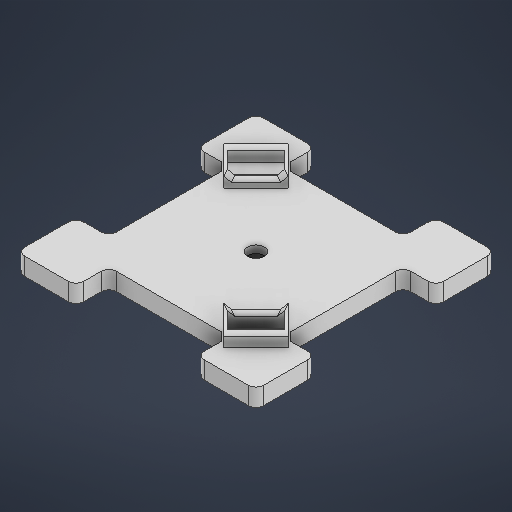
# Autodesk Inventor part: SistemaDeDesacople
Saved by Autodesk Inventor 2026.1 (Build 301233000, 233)
## iProperties
Created: 2026-01-17
Part Number: SistemaDeDesacople
Material: Genérico
Document SubType Name: Modeling
Designer: vickh
Density: 1 g/cm^3
Appearance: Valor por defecto
Author: vickh
Autodesk Inventor part; units mm, degrees
ref_plane "YZ Plane" through (0, 0, 0) normal (1, 0, 0) x (0, 1, 0)
ref_plane "XZ Plane" through (0, 0, 0) normal (0, 1, 0) x (-1, 0, 0)
ref_plane "XY Plane" through (0, 0, 0) normal (0, 0, 1) x (1, 0, 0)
sketch "Boceto1" plane through (0, 0, 0) normal (0, 1, 0) x (-1, 0, 0)
  line L0 (34.5, 0) -> (34.5, 24)
  line L1 (34.5, 24) -> (47.5, 24)
  line L2 (24, 47.5) -> (24, 34.5)
  line L3 (24, 34.5) -> (-24, 34.5)
  line L4 (-24, 34.5) -> (-24, 47.5)
  line L5 (-34.5, 24) -> (-47.5, 24)
  line L6 (47.5, 0) -> (-47.5, 0) construction
  line L7 (-47.5, 47.5) -> (-24, 47.5)
  line L8 (24, 47.5) -> (47.5, 47.5)
  line L9 (-47.5, 24) -> (-47.5, 47.5)
  line L10 (47.5, 47.5) -> (47.5, 24)
  line L11 (-34.5, 24) -> (-34.5, 0)
  line L12 (34.5, 0) -> (34.5, -24)
  line L13 (34.5, -24) -> (47.5, -24)
  line L14 (24, -47.5) -> (24, -34.5)
  line L15 (24, -34.5) -> (-24, -34.5)
  line L16 (-24, -34.5) -> (-24, -47.5)
  line L17 (-34.5, -24) -> (-47.5, -24)
  line L18 (-47.5, -47.5) -> (-24, -47.5)
  line L19 (24, -47.5) -> (47.5, -47.5)
  line L20 (-47.5, -24) -> (-47.5, -47.5)
  line L21 (47.5, -47.5) -> (47.5, -24)
  line L22 (-34.5, -24) -> (-34.5, 0)
  line L23 (-47.5, -47.5) -> (47.5, 47.5) construction
  line L24 (-47.5, 47.5) -> (47.5, -47.5) construction
  point P0 (0, 0)
  point P1 (0, -34.5)
  point P2 (24, 41)
  point P3 (0, 0)
  point P4 (35.75, 47.5)
  dimension "d0" = 95
  dimension "d9" = 13
  dimension "d10" = 23.5
  dimension "d15" = 23.5
  dimension "d71" = 95
  constraints: 50 end point, 10 symmetric about line, 6 perpendicular, 5 midpoint, 4 equal length, 3 vertical, 2 point on line, 1 coincident, 1 horizontal, 1 parallel
  measures "d0" distance of L7.start L8.end
  measures "d9" distance from line of L2.start L3
  measures "d10" distance between parallel lines of L9 L4
  measures "d15" distance of L5.end L7.start
  measures "d71" distance from line of point (35.75, 47.5) L19
extrude "Extrusión1" add sketch "Boceto1" along normal blind 7
chamfer "Chaflán4" distance 3.2 angle 45 4 edges at (24, 3.5, 34.5) (34.5, 3.5, 24) (-24, 3.5, -34.5) (-34.5, 3.5, -24)
sketch "Boceto2" plane through (0, 7, 0) normal (0, 1, 0) x (1, 0, 0)
  line L0 (-27.5, -27.5) -> (27.5, -27.5)
  line L1 (27.5, -27.5) -> (27.5, 27.5)
  line L2 (27.5, 27.5) -> (-27.5, 27.5)
  line L3 (-27.5, 27.5) -> (-27.5, -27.5)
  line L4 (-27.5, -27.5) -> (27.5, 27.5) construction
  line L5 (27.5, -27.5) -> (-27.5, 27.5) construction
  line L6 (-29.9749, 18.6612) -> (-18.6612, 29.9749)
  line L7 (-18.6612, 29.9749) -> (-25.0251, 36.3388)
  line L8 (-25.0251, 36.3388) -> (-36.3388, 25.0251)
  line L9 (-36.3388, 25.0251) -> (-29.9749, 18.6612)
  line L10 (-29.9749, 18.6612) -> (-25.0251, 36.3388) construction
  line L11 (-18.6612, 29.9749) -> (-36.3388, 25.0251) construction
  line L12 (-15.4792, 28.2071) -> (-26.7929, 39.5208)
  line L13 (-26.7929, 39.5208) -> (-39.5208, 26.7929)
  line L14 (-39.5208, 26.7929) -> (-28.2071, 15.4792)
  line L15 (-28.2071, 15.4792) -> (-15.4792, 28.2071)
  line L16 (-15.4792, 28.2071) -> (-39.5208, 26.7929) construction
  line L17 (-26.7929, 39.5208) -> (-28.2071, 15.4792) construction
  line L18 (-34.5, 24) -> (-34.5, -24) projected
  line L19 (-34.5, 0) -> (34.5, 0) construction
  line L20 (34.5, -24) -> (34.5, 24) projected
  line L21 (-18.6612, 29.9749) -> (-15.4792, 28.2071)
  line L22 (-29.9749, 18.6612) -> (-28.2071, 15.4792)
  line L23 (29.9749, -18.6612) -> (18.6612, -29.9749)
  line L24 (18.6612, -29.9749) -> (36.3388, -25.0251) construction
  line L25 (18.6612, -29.9749) -> (15.4792, -28.2071)
  line L26 (15.4792, -28.2071) -> (39.5208, -26.7929) construction
  line L27 (25.0251, -36.3388) -> (36.3388, -25.0251)
  line L28 (29.9749, -18.6612) -> (25.0251, -36.3388) construction
  line L29 (18.6612, -29.9749) -> (25.0251, -36.3388)
  line L30 (26.7929, -39.5208) -> (28.2071, -15.4792) construction
  line L31 (15.4792, -28.2071) -> (26.7929, -39.5208)
  line L32 (26.7929, -39.5208) -> (39.5208, -26.7929)
  line L33 (28.2071, -15.4792) -> (15.4792, -28.2071)
  line L34 (36.3388, -25.0251) -> (29.9749, -18.6612)
  line L35 (29.9749, -18.6612) -> (28.2071, -15.4792)
  line L36 (39.5208, -26.7929) -> (28.2071, -15.4792)
  point P0 (0, 0)
  point P1 (-27.5, 27.5)
  point P2 (27.5, -27.5)
  point P3 (27.5, -27.5)
  point P4 (34.5, -24)
  dimension "d21" = 55
  dimension "d22" = 55
  dimension "d23" = 16
  dimension "d24" = 9
  dimension "d25" = 18
  dimension "d26" = 16
  dimension "d51" = 135
  dimension "d52" = 135
  dimension "d55" = 360
  constraints: 70 end point, 11 midpoint, 6 parallel, 3 perpendicular, 2 horizontal, 51 other
  measures "d21" distance of L2.end L1.end
  measures "d22" distance of L1.end L0.end
  measures "d23" distance of L8.end L7.end
  measures "d24" distance of L7.end L6.end
  measures "d25" distance of L12.end L13.end
  measures "d26" distance of L13.end L14.end
  measures "d51" angle of L12 L2
  measures "d52" angle of L7 L2
sketch "Boceto3" plane through (0, 0, 0) normal (0, -1, 0) x (1, 0, 0)
  line L0 (47.5, 47.5) -> (47.5, 24) projected
  line L1 (47.5, 47.5) -> (24, 47.5)
  line L2 (24, 47.5) -> (24, 24)
  line L3 (24, 24) -> (47.5, 24)
  line L4 (47.5, 24) -> (47.5, 47.5)
  line L5 (24, 34.5) -> (24, 47.5) projected
  line L6 (47.5, 24) -> (34.5, 24) projected
  circle A0 centre (40.75, 40.75) radius 2.5
  line L7 (0, 48.9307) -> (0, -48.9307) construction
  line L8 (51.06, 0) -> (-51.06, 0) construction
  circle A1 centre (-40.75, 40.75) radius 2.5
  circle A2 centre (-40.75, -40.75) radius 2.5
  circle A3 centre (40.75, -40.75) radius 2.5
  line L9 (47.5, 47.5) -> (24, 24) construction
  line L10 (24, 47.5) -> (47.5, 24) construction
  point P0 (0, 0)
  point P1 (0, 0)
  point P2 (35.75, 35.75)
  dimension "d41" = 5
  dimension "d77" = 360
  dimension "d80" = 5
  constraints: 16 end point, 4 centre point, 3 midpoint, 2 collinear, 2 horizontal, 2 parallel, 1 coincident, 1 perpendicular, 1 point on line, 1 vertical, 9 other
  measures "d41" diameter of A0
  measures "d80" horizontal distance of A0.centre point (35.75, 35.75)
extrude "Extrusión6" cut sketch "Boceto3" against normal blind 4 contours A0 | A1 | A2 | A3
sketch "Boceto4" plane through (0, 7, 0) normal (0, 1, 0) x (1, 0, 0)
  circle A0 centre (0, 0) radius 3.3
  dimension "d44" = 6.6
  constraints: 1 centre point, 1 coincident
  measures "d44" diameter of A0
extrude "Extrusión7" cut sketch "Boceto4" against normal up to next
sketch "Boceto5" plane through (0, 0, 0) normal (0, -1, 0) x (1, 0, 0)
  circle A0 centre (0, 0) radius 6.5
  dimension "d47" = 13
  constraints: 1 centre point, 1 coincident
  measures "d47" diameter of A0
extrude "Extrusión8" cut sketch "Boceto5" against normal blind 4
extrude "Extrusión9" add sketch "Boceto2" along normal blind 4 contours L25 L29 L27 L34 L20 L36 L32 L31 | L14 L18 L9 L22 | L36 L20 L34 L35 | L14 L13 L12 L21 L7 L8 L9 L18
extrude "Extrusión10" add sketch "Boceto2" along normal blind 2 contours L33 L1 L23 L0 | L0 L23 L25 L33 | L15 L22 L6 L3 | L3 L6 L2 L15 | L33 L35 L23 L1 | L2 L6 L21 L15
chamfer "Chaflán3" distance 2 angle 45 4 edges at (-17.0702, 9, -29.091) (-29.091, 9, -17.0702) (29.091, 9, 17.0702) (17.0702, 9, 29.091)
sketch "Boceto7" plane through (0, 7, 0) normal (0, 1, 0) x (1, 0, 0)
  line L0 (20.7825, -32.0962) -> (32.0962, -20.7825)
  line L1 (32.0962, -20.7825) -> (29.9749, -18.6612)
  line L2 (29.9749, -18.6612) -> (18.6612, -29.9749)
  line L3 (18.6612, -29.9749) -> (20.7825, -32.0962)
  line L4 (20.7825, -32.0962) -> (29.9749, -18.6612) construction
  line L5 (32.0962, -20.7825) -> (18.6612, -29.9749) construction
  line L6 (20.132, -28.5041) -> (28.5041, -20.132) projected
  line L7 (18.6612, -29.9749) -> (25.0251, -36.3388) projected
  line L8 (-20.7825, 32.0962) -> (-32.0962, 20.7825)
  line L9 (-32.0962, 20.7825) -> (-29.9749, 18.6612)
  line L10 (-29.9749, 18.6612) -> (-18.6612, 29.9749)
  line L11 (-18.6612, 29.9749) -> (-20.7825, 32.0962)
  line L12 (-20.7825, 32.0962) -> (-29.9749, 18.6612) construction
  line L13 (-32.0962, 20.7825) -> (-18.6612, 29.9749) construction
  line L14 (36.3388, -25.0251) -> (29.9749, -18.6612) projected
  point P0 (0, 0)
  point P1 (25.3787, -25.3787)
  point P2 (-20.132, 28.5041)
  point P3 (-28.5041, 20.132)
  point P4 (-18.6612, 29.9749)
  point P5 (-25.3787, 25.3787)
  point P6 (33.5, -22.1863)
  dimension "d64" = 3
  dimension "d67" = 360
  constraints: 24 end point, 4 midpoint, 3 coincident, 3 collinear, 3 parallel, 1 perpendicular, 31 other
  measures "d64" distance between parallel lines of L0 L2
extrude "Extrusión11" cut sketch "Boceto7" against normal up to next
fillet "Empalme1" radius 3 16 edges at (24, 3.5, 47.5) (47.5, 3.5, 47.5) (47.5, 3.5, 24) (47.5, 3.5, -24) (34.5, 3.5, -24) (47.5, 3.5, -47.5) (24, 3.5, -47.5) (24, 3.5, -34.5) (-24, 3.5, -47.5) (-47.5, 3.5, -47.5) (-47.5, 3.5, -24) (-47.5, 3.5, 24) (-34.5, 3.5, 24) (-47.5, 3.5, 47.5) (-24, 3.5, 47.5) (-24, 3.5, 34.5)
equation "\"d15\" = d13"
equation "\"d13\" = 23.5"
